Make two of these (Autodesk Fusion 360 design; units mm, degrees)
Autodesk Fusion 360 part; units mm, degrees
sketch "Sketch1" plane through (0, 0, 0) normal (0, 1, 0) x (1, 0, 0)
  line L0 (0, 0) -> (76.2, 0)
  line L1 (76.2, 0) -> (76.2, 254)
  line L2 (76.2, 254) -> (0, 254)
  line L3 (0, 254) -> (0, 0)
  constraint horizontal L0
  constraint vertical L1
  constraint horizontal L2
  constraint vertical L3
  constraint coincident L0.start L3.end
extrude "Extrude1" add sketch "Sketch1" along normal blind 6.35
sketch "Sketch2" plane through (0, 6.35, 0) normal (0, 1, 0) x (-1, 0, 0)
  line L0 (0, -254) -> (0, 0)
  line L1 (0, 0) -> (-76.2, 0)
  line L2 (-76.2, 0) -> (-76.2, -254)
  line L3 (-76.2, -254) -> (0, -254)
  circle A0 centre (-25.4, -25.4) radius 1.27
  circle A1 centre (-50.8, -25.4) radius 1.27
  circle A2 centre (-25.4, -241.3) radius 1.27
  circle A3 centre (-50.8, -241.3) radius 1.27
  dimension "d3" = 2.54
  dimension "d4" = 2.54
  dimension "d5" = 2.54
  dimension "d6" = 2.54
  measures "d3" diameter of A0
  measures "d4" diameter of A1
  measures "d5" diameter of A2
  measures "d6" diameter of A3
extrude "Extrude2" cut sketch "Sketch2" against normal blind 6.35 contours A0
sketch "Sketch3" plane through (0, 6.35, 0) normal (0, 1, 0) x (-1, 0, 0)
  circle A0 centre (-25.4, -25.4) radius 1.27
  line L0 (0, -254) -> (0, 0)
  line L1 (0, 0) -> (-76.2, 0)
  line L2 (-76.2, 0) -> (-76.2, -254)
  line L3 (-76.2, -254) -> (0, -254)
  circle A1 centre (-50.8, -25.4) radius 1.27
  dimension "d9" = 2.54
  measures "d9" diameter of A1
extrude "Extrude3" cut sketch "Sketch3" against normal blind 6.35 contours A1
sketch "Sketch4" plane through (0, 6.35, 0) normal (0, 1, 0) x (-1, 0, 0)
  circle A0 centre (-50.8, -25.4) radius 1.27
  circle A1 centre (-25.4, -25.4) radius 1.27
  line L0 (0, -254) -> (0, 0)
  line L1 (0, 0) -> (-76.2, 0)
  line L2 (-76.2, 0) -> (-76.2, -254)
  line L3 (-76.2, -254) -> (0, -254)
  circle A2 centre (-25.4, -241.3) radius 1.27
  dimension "d12" = 2.54
  measures "d12" diameter of A2
extrude "Extrude4" cut sketch "Sketch4" against normal blind 6.35 contours A2
sketch "Sketch5" plane through (0, 6.35, 0) normal (0, 1, 0) x (-1, 0, 0)
  circle A0 centre (-25.4, -241.3) radius 1.27
  circle A1 centre (-50.8, -25.4) radius 1.27
  circle A2 centre (-25.4, -25.4) radius 1.27
  line L0 (0, -254) -> (0, 0)
  line L1 (0, 0) -> (-76.2, 0)
  line L2 (-76.2, 0) -> (-76.2, -254)
  line L3 (-76.2, -254) -> (0, -254)
  circle A3 centre (-50.8, -241.3) radius 1.27
  dimension "d15" = 2.54
  measures "d15" diameter of A3
extrude "Extrude5" cut sketch "Sketch5" against normal blind 6.35 contours A3
